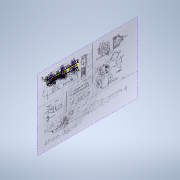
# Autodesk Inventor part: Part1
Saved by Autodesk Inventor 2021 (Build 250183000, 183)
## iProperties
Created: 2021-08-19
Part Number: Part1
Material: Generic
Document SubType Name: Modeling
Designer: newic
Density: 1 g/cm^3
Appearance: Default
Author: newic
Autodesk Inventor part; units mm, degrees
ref_plane "YZ Plane" through (0, 0, 0) normal (1, 0, 0) x (0, 1, 0)
ref_plane "XZ Plane" through (0, 0, 0) normal (0, 1, 0) x (-1, 0, 0)
ref_plane "XY Plane" through (0, 0, 0) normal (0, 0, 1) x (1, 0, 0)
sketch "Sketch1" plane through (0, 0, 0) normal (0, 1, 0) x (-1, 0, 0)
  line L0 (0, 0) -> (139.7, 0)
  line L1 (139.7, 0) -> (139.7, -920.75)
  line L2 (139.7, -920.75) -> (0, -920.75)
  line L3 (0, -920.75) -> (0, 0)
  dimension "d0" = 139.7
  dimension "d1" = 920.75
  constraints: 8 end point, 2 parallel, 1 horizontal, 1 perpendicular
  measures "d0" distance of L1.end L2.end
  measures "d1" distance of L0.end L1.end
extrude "Extrusion1" add sketch "Sketch1" along normal blind 100.33
sketch "Sketch2" plane through (0, 0, 0) normal (1, 0, 0) x (0, 0, -1)
  line L0 (920.75, 0) -> (0, 0) projected
  line L1 (0, 0) -> (920.75, 0)
  line L2 (-297.6389, 409.8513) -> (2710.7909, 409.8513) construction
  line L3 (2710.7909, 409.8513) -> (2710.7909, -1716.9746) construction
  line L4 (2710.7909, -1716.9746) -> (-297.6389, -1716.9746) construction
  line L5 (-297.6389, -1716.9746) -> (-297.6389, 409.8513) construction
  line L6 (0, 0) -> (920.75, 0) projected
  line L7 (920.75, 0) -> (920.75, 100.33) projected
  line L8 (0, 100.33) -> (920.75, 100.33) projected
  line L9 (0, 0) -> (0, 100.33) projected
  line L10 (0, 100.33) -> (0, 120.65)
  line L11 (0, 120.65) -> (920.75, 120.65)
  line L12 (920.75, 120.65) -> (920.75, 100.33)
  line L13 (0, 120.65) -> (0, 196.85)
  line L14 (920.75, 196.85) -> (920.75, 120.65)
  line L15 (477.9962, 0) -> (477.9962, -13.97)
  line L16 (477.9962, -13.97) -> (434.8162, -13.97)
  line L17 (434.8162, -13.97) -> (434.8162, 0)
  line L18 (133.294, 0) -> (133.294, -13.97)
  line L19 (133.294, -13.97) -> (90.114, -13.97)
  line L20 (90.114, -13.97) -> (90.114, 0)
  line L21 (769.0257, 0) -> (769.0257, -13.97)
  line L22 (769.0257, -13.97) -> (812.2057, -13.97)
  line L23 (812.2057, -13.97) -> (812.2057, 0)
  line L24 (434.8162, -13.97) -> (477.9962, -13.97)
  line L25 (769.0257, -13.97) -> (812.2057, -13.97)
  line L26 (90.114, -13.97) -> (133.294, -13.97)
  line L27 (90.114, -13.97) -> (111.704, -13.97)
  line L28 (111.704, -13.97) -> (100.909, -13.97)
  line L29 (100.909, -13.97) -> (122.499, -13.97)
  line L30 (122.499, -13.97) -> (122.499, -33.02)
  line L31 (122.499, -33.02) -> (100.909, -33.02)
  line L32 (100.909, -33.02) -> (100.909, -13.97)
  line L33 (434.8162, -13.97) -> (456.4062, -13.97)
  line L34 (456.4062, -13.97) -> (445.6112, -13.97)
  line L35 (445.6112, -13.97) -> (467.2012, -13.97)
  line L36 (467.2012, -13.97) -> (467.2012, -33.02)
  line L37 (467.2012, -33.02) -> (445.6112, -33.02)
  line L38 (445.6112, -33.02) -> (445.6112, -13.97)
  line L39 (769.0257, -13.97) -> (790.6157, -13.97)
  line L40 (790.6157, -13.97) -> (779.8207, -13.97)
  line L41 (779.8207, -13.97) -> (801.4107, -13.97)
  line L42 (801.4107, -13.97) -> (801.4107, -33.02)
  line L43 (801.4107, -33.02) -> (779.8207, -33.02)
  line L44 (779.8207, -33.02) -> (779.8207, -13.97)
  line L45 (434.8162, 0) -> (413.2262, 0)
  line L46 (413.2262, 0) -> (413.2262, -11.43)
  line L47 (413.2262, -11.43) -> (371.9512, -11.43)
  line L48 (371.9512, -11.43) -> (371.9512, 64.77)
  arc A0 (413.2262, 72.0379) -> (371.9512, 72.0379) centre (392.5887, 68.404) ccw
  line L49 (413.2262, 0) -> (413.2262, 64.77)
  line L50 (371.9512, 64.77) -> (371.9512, 72.0379)
  line L51 (413.2262, 64.77) -> (413.2262, 72.0379)
  line L52 (434.8162, -13.97) -> (434.8162, 202.565)
  line L53 (477.9962, -13.97) -> (477.9962, 202.565)
  line L54 (769.0257, -13.97) -> (769.0257, 202.565)
  line L55 (812.2057, -13.97) -> (812.2057, 202.565)
  line L56 (812.2057, 202.565) -> (769.0257, 202.565)
  line L57 (477.9962, 202.565) -> (434.8162, 202.565)
  line L58 (133.294, -13.97) -> (133.294, 182.245)
  line L59 (90.114, -13.97) -> (90.114, 182.245)
  line L60 (90.114, 182.245) -> (133.294, 182.245)
  line L61 (67.3834, 182.245) -> (164.6776, 182.245)
  line L62 (413.2262, 202.565) -> (508.4774, 202.565)
  line L63 (745.5808, 202.565) -> (847.3717, 202.565)
  line L64 (67.3834, 161.925) -> (164.6776, 161.925)
  line L65 (413.2262, 182.245) -> (508.4774, 182.245)
  line L66 (745.5808, 182.245) -> (847.3717, 182.245)
  line L67 (133.294, -13.97) -> (133.294, 78.74)
  line L68 (133.294, 78.74) -> (434.8162, 78.74)
  line L69 (133.294, -13.97) -> (133.294, 26.67)
  line L70 (133.294, 26.67) -> (371.9512, 26.67)
  line L71 (133.294, 26.67) -> (298.394, 26.67)
  line L72 (298.394, 26.67) -> (317.7759, 78.74)
  line L73 (133.294, 78.74) -> (133.294, 59.055)
  line L74 (133.294, 59.055) -> (310.4486, 59.055)
  dimension "d4" = 920.75
  dimension "d32" = 20.32
  dimension "d33" = 76.2
  dimension "d34" = 13.97
  dimension "d35" = 43.18
  dimension "d36" = 13.97
  dimension "d37" = 43.18
  dimension "d38" = 13.97
  dimension "d39" = 13.97
  dimension "d40" = 43.18
  dimension "d45" = 21.59
  dimension "d46" = 19.05
  dimension "d47" = 21.59
  dimension "d48" = 19.05
  dimension "d49" = 21.59
  dimension "d50" = 19.05
  dimension "d58" = 21.59
  dimension "d59" = 11.43
  dimension "d60" = 41.275
  dimension "d61" = 76.2
  dimension "d63" = 20.955
  dimension "d65" = 216.535
  dimension "d66" = 216.535
  dimension "d67" = 216.535
  dimension "d68" = 216.535
  dimension "d69" = 196.215
  dimension "d71" = 20.32
  dimension "d72" = 20.32
  dimension "d73" = 20.32
  dimension "d74" = 92.71
  dimension "d75" = 40.64
  dimension "d76" = 165.1
  dimension "d77" = 19.685
  constraints: 132 end point, 14 perpendicular, 12 horizontal, 11 point on line, 11 vertical, 10 equal length, 7 midpoint, 2 point on circle, 1 centre point, 10 other
  measures "d4" distance of L0.start L0.end
  measures "d32" distance of L8.start L10.end
  measures "d33" distance of L10.end L13.end
  measures "d34" distance of L15.start L15.end
  measures "d35" distance of L15.end L16.end
  measures "d36" distance of L18.start L18.end
  measures "d37" distance of L18.end L19.end
  measures "d38" distance of L19.end L20.end
  measures "d39" distance of L21.start L21.end
  measures "d40" distance of L21.end L22.end
  measures "d45" distance of L30.end L31.end
  measures "d46" distance of L29.end L30.end
  measures "d47" distance of L36.end L37.end
  measures "d48" distance of L35.end L36.end
  measures "d49" distance of L42.end L43.end
  measures "d50" distance of L41.end L42.end
  measures "d58" distance of L17.end L45.end
  measures "d59" distance of L45.end L46.end
  measures "d60" distance of L46.end L47.end
  measures "d61" distance of L47.end L48.end
  measures "d63" radius of A0
  measures "d65" distance of L16.end L52.end
  measures "d66" distance of L24.end L53.end
  measures "d67" distance of L21.end L54.end
  measures "d68" distance of L25.end L55.end
  measures "d69" distance of L26.end L58.end
  measures "d71" distance between parallel lines of L61 L64
  measures "d72" distance between parallel lines of L62 L65
  measures "d73" distance between parallel lines of L63 L66
  measures "d74" distance of L26.end L67.end
  measures "d75" distance of L26.end L69.end
  measures "d76" distance of L69.end L71.end
  measures "d77" distance of L67.end L73.end
body "Solid1"
